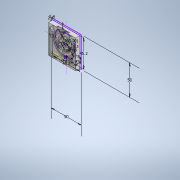
# Autodesk Inventor part: BaseCharger
Saved by Autodesk Inventor 2022 (Build 260153000, 153)
## iProperties
Created: 2022-08-22
Part Number: BaseCharger
Material: Generic
Document SubType Name: Modeling
Designer: sgioj
Density: 1 g/cm^3
Appearance: Default
Author: sgioj
Autodesk Inventor part; units mm, degrees
ref_plane "YZ Plane" through (0, 0, 0) normal (1, 0, 0) x (0, 1, 0)
ref_plane "XZ Plane" through (0, 0, 0) normal (0, 1, 0) x (-1, 0, 0)
ref_plane "XY Plane" through (0, 0, 0) normal (0, 0, 1) x (1, 0, 0)
sketch "Sketch1" plane through (-19.533607, 25, 0) normal (0, 0, 1) x (1, 0, 0)
  line L0 (0, 0) -> (50, 0)
  line L1 (50, 0) -> (50, -50)
  line L2 (50, -50) -> (0, -50)
  line L3 (0, -50) -> (0, 0)
  line L4 (2.4, -2.4) -> (47.6, -2.4)
  line L5 (47.6, -2.4) -> (47.6, -47.6)
  line L6 (47.6, -47.6) -> (2.4, -47.6)
  line L7 (2.4, -47.6) -> (2.4, -2.4)
  line L8 (2.4, -2.4) -> (47.6, -47.6) construction
  line L9 (47.6, -2.4) -> (2.4, -47.6) construction
  circle A0 centre (25, -25) radius 19.375
  circle A1 centre (25, -25) radius 14.5
  circle A2 centre (25, -25) radius 4.175
  circle A3 centre (31.679764, -18.320236) radius 2.65
  circle A4 centre (25, -15.553387) radius 2.65
  circle A5 centre (18.320236, -18.320236) radius 2.65
  circle A6 centre (15.553387, -25) radius 2.65
  circle A7 centre (18.320236, -31.679764) radius 2.65
  circle A8 centre (25, -34.446613) radius 2.65
  circle A9 centre (31.679764, -31.679764) radius 2.65
  circle A10 centre (34.446613, -25) radius 2.65
  line L10 (50, -25) -> (-10.932785, -25) construction
  line L11 (33.553597, -16.446403) -> (35.253048, -14.746952)
  line L12 (33.553597, -33.553597) -> (35.253048, -35.253048)
  arc A11 (16.446403, -16.446403) -> (16.447482, -33.554675) centre (24.992317, -25) ccw
  line L13 (16.446403, -16.446403) -> (14.746952, -14.746952)
  line L14 (16.447482, -33.554675) -> (14.746952, -35.253048)
  line L15 (3.4, -3.4) -> (46.6, -3.4)
  line L16 (46.6, -3.4) -> (46.6, -46.6)
  line L17 (46.6, -46.6) -> (3.4, -46.6)
  line L18 (3.4, -46.6) -> (3.4, -3.4)
  line L19 (46.6, -46.6) -> (43.6, -46.6)
  line L20 (43.6, -46.6) -> (43.6, -43.6)
  line L21 (43.6, -43.6) -> (46.6, -43.6)
  line L22 (46.6, -43.6) -> (46.6, -46.6)
  line L23 (43.6, -43.6) -> (38.700194, -43.6)
  line L24 (38.700194, -43.6) -> (38.700194, -38.700194)
  line L25 (38.700194, -38.700194) -> (43.6, -38.700194)
  line L26 (43.6, -38.700194) -> (43.6, -43.6)
  line L27 (43.6, -38.700194) -> (46.6, -38.700194)
  line L28 (46.6, -38.700194) -> (46.6, -35.700194)
  line L29 (46.6, -35.700194) -> (43.6, -35.700194)
  line L30 (43.6, -35.700194) -> (43.6, -38.700194)
  line L31 (46.6, -35.700194) -> (42.820879, -35.700194)
  line L32 (42.820879, -35.700194) -> (42.820879, -32.603085)
  line L33 (42.820879, -32.603085) -> (46.6, -32.603085)
  line L34 (46.6, -32.603085) -> (46.6, -35.700194)
  line L35 (38.700194, -43.6) -> (35.700194, -43.6)
  line L36 (35.700194, -43.6) -> (35.700194, -46.6)
  line L37 (35.700194, -46.6) -> (38.700194, -46.6)
  line L38 (38.700194, -46.6) -> (38.700194, -43.6)
  line L39 (35.700194, -46.6) -> (32.383701, -46.6)
  line L40 (32.383701, -46.6) -> (32.383701, -42.912889)
  line L41 (32.383701, -42.912889) -> (35.700194, -42.912889)
  line L42 (35.700194, -42.912889) -> (35.700194, -46.6)
  line L43 (23.5, -43.2) -> (26.5, -43.2)
  line L44 (26.5, -43.2) -> (26.5, -50)
  line L45 (26.5, -50) -> (23.5, -50)
  line L46 (23.5, -50) -> (23.5, -43.2)
  line L47 (23.5, -43.2) -> (26.5, -50) construction
  line L48 (26.5, -43.2) -> (23.5, -50) construction
  circle A12 centre (7.947368, -7.947368) radius 4.547368
  circle A13 centre (42.052632, -7.947368) radius 4.547368
  line L49 (2.4, -47.6) -> (2.4, -50)
  line L50 (47.6, -47.6) -> (47.6, -50)
  line L51 (22.407108, -14.233364) -> (20.194069, -16.446403)
  line L52 (25, 8.52179) -> (25, -70.2) construction
  line L53 (18.320236, -8.83287) -> (18.320236, -33.554675) construction
  line L54 (18.320236, -14.57257) -> (20.194069, -16.446403)
  line L55 (18.320236, -14.57257) -> (20.533275, -12.359531)
  line L56 (22.407108, -14.233364) -> (20.533275, -12.359531)
  line L57 (18.320236, -14.57257) -> (19.593028, -13.299778)
  line L58 (19.593028, -13.299778) -> (20.86582, -14.57257)
  line L59 (20.86582, -14.57257) -> (19.593028, -15.845362)
  line L60 (27.592892, -14.233364) -> (29.805931, -16.446403)
  line L61 (31.679764, -14.57257) -> (29.805931, -16.446403)
  line L62 (31.679764, -14.57257) -> (29.466725, -12.359531)
  line L63 (27.592892, -14.233364) -> (29.466725, -12.359531)
  line L64 (20.194069, -16.446403) -> (22.407108, -14.233364)
  line L65 (22.407108, -14.233364) -> (22.601124, -14.42738)
  line L66 (22.601124, -14.42738) -> (20.388085, -16.640419)
  line L67 (20.388085, -16.640419) -> (20.194069, -16.446403)
  line L68 (30.406972, -13.299778) -> (29.13418, -14.57257)
  line L69 (29.13418, -14.57257) -> (30.406972, -15.845362)
  line L70 (27.592892, -14.233364) -> (27.398876, -14.42738)
  line L71 (27.398876, -14.42738) -> (29.611915, -16.640419)
  line L72 (29.611915, -16.640419) -> (29.805931, -16.446403)
  line L73 (22.407108, -14.233364) -> (20.533275, -12.359531)
  line L74 (20.533275, -12.359531) -> (21.735357, -11.157449)
  line L75 (21.735357, -11.157449) -> (23.60919, -13.031282)
  line L76 (23.60919, -13.031282) -> (22.407108, -14.233364)
  line L77 (29.466725, -12.359531) -> (28.264643, -11.157449)
  line L78 (28.264643, -11.157449) -> (26.39081, -13.031282)
  line L79 (26.39081, -13.031282) -> (27.592892, -14.233364)
  point P0 (25, -46.6)
  point P1 (26.5, -44.316848)
  point P2 (26.5, -46.6)
  point P3 (42.052632, -3.4)
  point P4 (46.6, -7.947368)
  point P5 (3.4, -7.947368)
  point P6 (7.947368, -3.4)
  point P7 (26.5, -47.6)
  point P8 (23.5, -47.6)
  dimension "d9" = 5.3
  dimension "d17" = 50
  dimension "d18" = 50
  dimension "d15" = 45.2
  dimension "d16" = 45.2
  dimension "d12" = 38.75
  dimension "d11" = 29
  dimension "d10" = 8.35
  dimension "d5" = 360
  dimension "d13" = 2.4
  dimension "d14" = 2.4
  dimension "d29" = 1
  dimension "d30" = 1
  dimension "d31" = 1
  dimension "d34" = 3
  dimension "d35" = 3
  dimension "d36" = 3
  dimension "d37" = 3
  dimension "d38" = 3
  dimension "d39" = 3
  dimension "d40" = 3
  dimension "d79" = 1.8
  dimension "d87" = 1.7
  constraints: 158 end point, 24 parallel, 17 perpendicular, 12 point on line, 11 centre point, 11 horizontal, 11 point on circle, 11 symmetric about line, 5 coincident, 5 midpoint, 2 tangent, 2 vertical, 39 other
  measures "d17" distance of L1.end L2.end
  measures "d18" distance of L0.end L1.end
  measures "d15" distance of L5.end L6.end
  measures "d16" distance of L4.end L5.end
  measures "d12" diameter of A0
  measures "d11" diameter of A1
  measures "d10" diameter of A2
  measures "d13" distance between parallel lines of L3 L7
  measures "d14" distance between parallel lines of L0 L4
  measures "d29" distance between parallel lines of L15 L4
  measures "d30" distance between parallel lines of L7 L18
  measures "d31" distance between parallel lines of L17 L6
  measures "d34" distance of L20.end L21.end
  measures "d35" distance of L19.end L20.end
  measures "d36" distance of L29.end L28.end
  measures "d37" distance of L28.end L27.end
  measures "d38" distance of L37.end L36.end
  measures "d39" distance of L36.end L35.end
  measures "d40" distance of L44.end L45.end
  measures "d79" distance of L54.start L57.end
  measures "d87" distance of L55.end L74.end
extrude "Extrusion1" add sketch "Sketch1" along normal blind 4 contours A1 L14 A11 A5 L67 L66 A4 L71 L72 A3 L11 | L11 A3 L61 L62 L77 L78 L79 L70 A4 L65 L76 L75 L74 L55 L54 A5 L13 A1 | L13 A11 L14 A1 | L72 L71 L70 L60 | L60 L63 L62 L68 L69 L61 | L54 L59 L58 L55 L56 L51 | L51 L65 L66 L67 | L79 L78 L77 L63 | L69 L68 L62 L61 | L56 L74 L75 L76 | L54 L55 L58 L59
extrude "Extrusion2" add sketch "Sketch1" against normal blind 0.2 contours L7 L4 L5 L6 L44 L17 L16 L15 L18 L46 | L46 L17 L44 L6 | L46 A0 L44 L17 | L17 L18 A12 L15 A13 L16 L33 A0 L46 | L44 A0 L40 L17 | L46 L43 L44 A0 | A0 L44 L43 L46 | L40 L41 L42 L36 L17 | L18 L15 A12 | A12 | L36 L35 L38 L17 | A0 L24 L35 L42 L41 | L32 L31 L30 L25 A0 | L33 L16 L29 L31 L32 | L38 L23 L20 L17 | L25 L26 L23 L24 | L15 L16 A13 | A13 | L20 L21 L16 L17 | L27 L16 L21 L26 | L30 L29 L16 L27 | A7 | A1 L14 A11 A5 L67 L66 A4 L71 L72 A3 L11 | L11 A3 L61 L62 L77 L78 L79 L70 A4 L65 L76 L75 L74 L55 L54 A5 L13 A1 | L13 A11 L14 A1 | A3 | A5 | L72 L71 L70 L60 | L60 L63 L62 L68 L69 L61 | L54 L59 L58 L55 L56 L51 | L51 L65 L66 L67 | L79 L78 L77 L63 | L69 L68 L62 L61 | L56 L74 L75 L76 | L54 L55 L58 L59 | A4 | A2 | A6 | A8 | A9 | A10
extrude "Extrusion3" add sketch "Sketch1" along normal blind 2 contours L7 L4 L5 L6 L44 L17 L16 L15 L18 L46 | L46 L17 L44 L6 | L46 A0 L44 L17 | L17 L18 A12 L15 A13 L16 L33 A0 L46 | L44 A0 L40 L17 | L40 L41 L42 L36 L17 | L18 L15 A12 | A12 | L36 L35 L38 L17 | A0 L24 L35 L42 L41 | L32 L31 L30 L25 A0 | L33 L16 L29 L31 L32 | L38 L23 L20 L17 | L25 L26 L23 L24 | L15 L16 A13 | A13 | L20 L21 L16 L17 | L27 L16 L21 L26 | L30 L29 L16 L27
extrude "Extrusion5" add sketch "Sketch1" along normal blind 7 contours L7 L4 L5 L6 L44 L17 L16 L15 L18 L46 | L46 L17 L44 L6
extrude "Extrusion6" add sketch "Sketch1" along normal blind 7 contours L44 A0 L40 L17 | L40 L41 L42 L36 L17 | L33 L16 L29 L31 L32 | L25 L26 L23 L24
sketch "Sketch3" plane through (-19.533607, 25, 2) normal (0, 0, 1) x (1, 0, 0)
  line L0 (23.5, -43.188515) -> (26.5, -43.188515)
  line L1 (26.5, -43.188515) -> (26.5, -50.011485)
  line L2 (26.5, -50.011485) -> (23.5, -50.011485)
  line L3 (23.5, -50.011485) -> (23.5, -43.188515)
  line L4 (26.5, -46.6) -> (3.4, -46.6)
  line L5 (23.5, -43.188515) -> (26.5, -50.011485) construction
  line L6 (26.5, -43.188515) -> (23.5, -50.011485) construction
  point P0 (19.533607, -25)
  point P1 (25, -46.6)
  point P2 (32.383701, -46.6)
  dimension "d43" = 3
  constraints: 12 end point, 2 midpoint, 2 parallel, 1 horizontal, 1 perpendicular, 1 point on line
  measures "d43" distance of L1.end L2.end
extrude "Extrusion10" add sketch "Sketch1" along normal blind 7 contours L49 L6 L46 L2 | L2 L44 L6 L50 | L46 L6 L44 L2
sketch "Sketch2" plane through (5.466393, 0, 4) normal (0, 0, 1) x (1, 0, 0)
  line L0 (-22.6, -22.6) -> (22.6, -22.6)
  line L1 (-9.773009, -2.851634) -> (-22.6, -2.851634)
  line L2 (-22.6, -2.851634) -> (-22.6, -22.6)
  line L3 (-22.6, -22.6) -> (-9.773009, -22.6)
  line L4 (-9.773009, -22.6) -> (-9.773009, -2.851634)
  line L5 (-9.773009, -22.6) -> (-22.6, -22.6)
  line L6 (-22.6, -22.6) -> (-22.6, -23.8)
  line L7 (-22.6, -23.8) -> (-9.773009, -23.8)
  line L8 (-9.773009, -23.8) -> (-9.773009, -22.6)
  line L9 (-21.6, 21.6) -> (-21.6, -21.6)
  line L10 (-21.6, -2.851634) -> (-21.6, -23.8)
  point P0 (-5.466393, 0)
  point P1 (-9.773009, -22.6)
  dimension "d63" = 19.74837
  dimension "d74" = 1.2
  constraints: 18 end point, 4 parallel, 3 perpendicular, 3 point on line, 2 horizontal
  measures "d63" distance between parallel lines of L0 L1
  measures "d74" distance of L6.end L5.end
sketch "Sketch4" plane through (-19.533607, 25, 7) normal (0, 0, 1) x (1, 0, 0)
  line L0 (23.5, -43.6) -> (26.5, -43.6)
  line L1 (26.5, -43.6) -> (26.5, -51.6)
  line L2 (26.5, -51.6) -> (23.5, -51.6)
  line L3 (23.5, -51.6) -> (23.5, -43.6)
  line L4 (2.4, -47.6) -> (47.6, -47.6) projected
  line L5 (23.5, -43.6) -> (26.5, -51.6) construction
  line L6 (26.5, -43.6) -> (23.5, -51.6) construction
  point P0 (19.533607, -25)
  point P1 (25, -47.6)
  point P2 (23.5, -47.6)
  point P3 (26.5, -47.6)
  dimension "d48" = 3
  dimension "d49" = 8
  constraints: 12 end point, 3 midpoint, 2 parallel, 1 horizontal, 1 perpendicular
  measures "d48" distance of L1.end L2.end
  measures "d49" distance of L0.end L1.end
extrude "Extrusion8" cut sketch "Sketch4" against normal blind 3.5
extrude "Extrusion9" add sketch "Sketch1" along normal blind 7 contours L18 L15 A12 | A12 | L15 L16 A13 | A13
hole "Hole1" at (-11.586239, 17.052632, 0) at (22.519024, 17.052632, 0) direction (0, 0, 1) diameter 4.915 end through all clearance for "Flat Head Machine Screw (82)" size "#8" standard "Ansi Unified Screw Threads"
hole "Hole2" at (-11.586239, 17.052632, 0) at (22.519024, 17.052632, 0) direction (0, 0, -1) diameter 4.915 end through all clearance for "Flat Head Machine Screw (82)" size "#8" standard "Ansi Unified Screw Threads"
chamfer "Chamfer1" distance 2 angle 45 2 edges at (-11.5862, 19.5101, -0.2) (22.519, 19.5101, -0.2) measured on face at (10.6074, -9.9956, -0.2)
extrude "Extrusion11" cut sketch "Sketch2" along normal blind 3 and the other way blind 2 contours L10 L9 L1 L4 L0 | L0 L8 L7 L10
extrude "Extrusion12" add sketch "Sketch1" along normal up to surface (7 mm away) contours L72 L71 L70 L60 | L60 L63 L62 L68 L69 L61 | L54 L59 L58 L55 L56 L51 | L51 L65 L66 L67 | L79 L78 L77 L63 | L56 L74 L75 L76
sketch "Sketch5" plane through (-17.133607, 22.6, -0.2) normal (0, 1, 0) x (1, 0, 0)
  point P0 (17.133607, -0.2)
sketch "Sketch6" plane through (-17.133607, 22.6, -0.2) normal (0, 1, 0) x (1, 0, 0)
  line L0 (17.794069, -7.2) -> (17.193028, -7.2)
  line L1 (17.794069, -7.2) -> (12.794069, -7.2)
  line L2 (12.794069, -7.2) -> (12.794069, -4.2)
  line L3 (12.794069, -4.2) -> (17.794069, -4.2)
  line L4 (17.794069, -4.2) -> (17.794069, -7.2)
  line L5 (28.006972, -7.2) -> (27.211915, -7.2)
  line L6 (34.696613, -4.2) -> (29.396613, -4.2)
  line L7 (27.405931, -7.2) -> (32.405931, -7.2)
  line L8 (32.405931, -7.2) -> (32.405931, -4.2)
  line L9 (32.405931, -4.2) -> (27.405931, -4.2)
  line L10 (27.405931, -4.2) -> (27.405931, -7.2)
  line L11 (27.405931, -4.2) -> (25.192892, -4.2)
  line L12 (27.405931, -4.2) -> (17.794069, -4.2)
  line L13 (17.794069, -7.2) -> (27.405931, -7.2)
  line L14 (17.193028, -4.2) -> (18.133275, -4.2)
  point P0 (17.133607, -0.2)
  point P1 (15.920236, -7.2)
  point P2 (29.279764, -7.2)
  point P3 (15.920236, -4.2)
  point P4 (17.193028, -7.2)
  dimension "d82" = 5
  dimension "d83" = 3
  dimension "d84" = 5
  constraints: 20 end point, 5 parallel, 2 horizontal, 2 perpendicular, 1 point on line
  measures "d82" distance of L2.end L3.end
  measures "d83" distance of L1.end L2.end
  measures "d84" distance of L9.end L8.end
extrude "Extrusion13" cut sketch "Sketch6" against normal up to next
body "Solid1"
